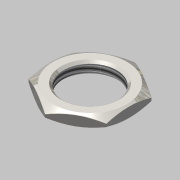
# Autodesk Inventor part: InputJack_nut
Saved by Autodesk Inventor 2015 SP1 (Build 190203100, 203)
## iProperties
Created: 2015-06-13
Part Number: InputJack_nut
Material: Generic
Document SubType Name: Modeling
Designer: Peter Mulkers
Density: 1 g/cm^3
Appearance: Titanium
Author: Peter Mulkers
Autodesk Inventor part; units mm, degrees
ref_plane "YZ Plane" through (0, 0, 0) normal (1, 0, 0) x (0, 1, 0)
ref_plane "XZ Plane" through (0, 0, 0) normal (0, 1, 0) x (-1, 0, 0)
ref_plane "XY Plane" through (0, 0, 0) normal (0, 0, 1) x (1, 0, 0)
sketch "Sketch1" plane through (0, 0, 0) normal (0, 0, 1) x (1, 0, 0)
  line L0 (6.35, -3.6662) -> (0, -7.3323)
  line L1 (0, -7.3323) -> (-6.35, -3.6662)
  line L2 (-6.35, -3.6662) -> (-6.35, 3.6662)
  line L3 (-6.35, 3.6662) -> (0, 7.3323)
  line L4 (0, 7.3323) -> (6.35, 3.6662)
  line L5 (6.35, 3.6662) -> (6.35, -3.6662)
  point P0 (0, 0)
  point P1 (0, 0)
  dimension "d0" = 12.7
  constraints: 12 end point, 1 coincident, 13 other
  measures "d0" distance between parallel lines of L5 L2
extrude "Extrusion1" add sketch "Sketch1" along normal blind 2
sketch "Sketch2" plane through (0, 0, 2) normal (0, 0, 1) x (1, 0, 0)
  point P0 (0, 0)
  point P1 (0, 0)
  constraints: 1 coincident
hole "Hole1" at (0, 0, 2) direction (0, 0, -1) diameter 8.661 end through all thread size "3/8-32 UNEF" class "2B" standard "ANSI Unified Screw Threads"
sketch "Sketch5" plane through (0, 0, 0) normal (1, 0, 0) x (0, 1, 0)
  line L0 (3.6662, 0) -> (7.3323, 0) construction
  line L1 (3.6662, 0) -> (3.6662, 2) construction
  line L2 (7.3323, 2) -> (3.6662, 2) construction
  line L3 (7.3323, 0) -> (7.3323, 2) construction
  line L4 (7.3323, 0) -> (6, 0)
  line L5 (6, 0) -> (7.3323, 0.7692)
  line L6 (7.3323, 0) -> (7.3323, 0.7692)
  line L7 (0, -0.4) -> (0, 2.4) projected
  line L8 (7.3323, 2) -> (7.3323, 1.2308)
  line L9 (7.3323, 1.2308) -> (6, 2)
  line L10 (6, 2) -> (7.3323, 2)
  point P0 (0, 0)
  dimension "d11" = 6
  dimension "d12" = 30
  dimension "d14" = 30
  constraints: 12 end point, 4 point on line, 2 collinear, 1 vertical alignment
  measures "d11" distance of point (0, 0) L4.end
  measures "d12" angle of L0 L5
  measures "d14" angle of L2 L9
revolve "Revolution1" cut sketch "Sketch5" angle 360 about axis through (0, 0, -10) along (0, 0, 1)
chamfer "Chamfer1" distance 0.375 angle 45 2 edges at (0, 4.3305, 0) (0, 4.3305, 2)
fillet "Fillet1" radius 0.1 22 edges at (6.35, -3.6662, 1) (6.35, 0, 1.7979) (6.35, 0, 0.2021) (6.35, 3.6662, 1) (3.175, 5.4993, 1.7979) (3.175, 5.4993, 0.2021) (0, 7.3323, 1) (-3.175, 5.4993, 1.7979) (-3.175, 5.4993, 0.2021) (-6.35, 3.6662, 1) (-6.35, 0, 0.2021) (-6.35, 0, 1.7979) (-6.35, -3.6662, 1) (-3.175, -5.4993, 1.7979) (-3.175, -5.4993, 0.2021) (0, -7.3323, 1) (3.175, -5.4993, 0.2021) (3.175, -5.4993, 1.7979) (0, -6, 2) (0, -6, 0) (0, 4.7055, 0) (0, 4.7055, 2)
body "Solid1"
